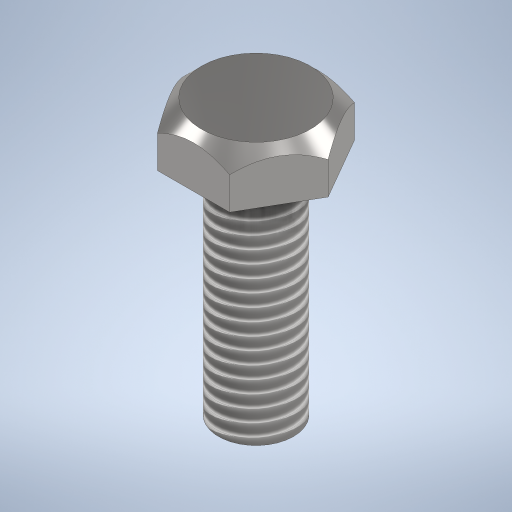
# Autodesk Inventor part: Tornillo
Saved by Autodesk Inventor 2023 (Build 270158000, 158)
## iProperties
Created: 2023-03-19
Part Number: Tornillo
Material: Acero inoxidable
Document SubType Name: Modeling
Designer: sergi
Density: 8 g/cm^3
Appearance: Semipulido
Author: sergi
Autodesk Inventor part; units mm, degrees
ref_plane "YZ Plane" through (0, 0, 0) normal (1, 0, 0) x (0, 1, 0)
ref_plane "XZ Plane" through (0, 0, 0) normal (0, 1, 0) x (-1, 0, 0)
ref_plane "XY Plane" through (0, 0, 0) normal (0, 0, 1) x (1, 0, 0)
sketch "Boceto1" plane through (0, 0, 0) normal (0, 1, 0) x (-1, 0, 0)
  point P0 (0, 0)
sketch "Boceto2" plane through (0, 0, 0) normal (0, 1, 0) x (-1, 0, 0)
  line L0 (1.4434, -2.5) -> (-1.4434, -2.5)
  line L1 (-1.4434, -2.5) -> (-2.8868, 0)
  line L2 (-2.8868, 0) -> (-1.4434, 2.5)
  line L3 (-1.4434, 2.5) -> (1.4434, 2.5)
  line L4 (1.4434, 2.5) -> (2.8868, 0)
  line L5 (2.8868, 0) -> (1.4434, -2.5)
  point P0 (0, 0)
  point P1 (0, 0)
  dimension "d0" = 5
  constraints: 12 end point, 1 coincident, 1 horizontal, 13 other
  measures "d0" distance between parallel lines of L2 L5
extrude "Extrusión1" add sketch "Boceto2" along normal blind 2
sketch "Boceto3" plane through (0, 0, 0) normal (0, -1, 0) x (1, 0, 0)
  circle A0 centre (0, 0) radius 1.5
  dimension "d3" = 3
  constraints: 1 centre point, 1 coincident
  measures "d3" diameter of A0
extrude "Extrusión2" add sketch "Boceto3" along normal blind 9
sketch "Boceto4" plane through (0, 0, 0) normal (0, 0, 1) x (1, 0, 0)
  line L0 (-2.8868, 0) -> (-2.8868, 2) projected
  line L1 (-2.8868, 1.3) -> (-2.8868, 2)
  line L2 (-2.8868, 2) -> (-2.1868, 2)
  line L3 (-2.8868, 2) -> (-1.4434, 2) projected
  line L4 (-2.8868, 1.3) -> (-2.1868, 2)
  line L5 (0, -11.2) -> (0, 4.2) projected
  point P0 (0, 0)
  dimension "d6" = 0.7
  dimension "d7" = 0.7
  constraints: 6 end point, 2 point on line, 1 vertical
  measures "d6" distance of L0.end L2.end
  measures "d7" distance of L0.end L1.start
revolve "Revolución1" cut sketch "Boceto4" angle 360 about axis through (0, -10, 0) along (0, 1, 0)
thread "Rosca1" size "M3x0.5" class "6g" standard "ISO Metric profile" full length
